Autodesk Inventor part; units mm, degrees
(part 2 of 2)
  spline S149 degree 2 poles (54.1022, 10.347) (54.1022, 11.4938) (55.3529, 12.7939) (56.4799, 12.7939) knots 0 0 0 1 2 2 2
  spline S150 degree 2 poles (56.4799, 12.7939) (57.607, 12.7939) (58.8527, 11.4889) (58.8527, 10.347) knots 0 0 0 1 2 2 2
  spline S151 degree 2 poles (57.3845, 10.3371) (57.3845, 10.7474) (57.2511, 11.2961) (57.1324, 11.4592) knots 0 0 0 1 2 2 2
  spline S152 degree 2 poles (57.1324, 11.4592) (57.0039, 11.6322) (56.6826, 11.7657) (56.4799, 11.7657) knots 0 0 0 1 2 2 2
  spline S153 degree 2 poles (56.4799, 11.7657) (56.2822, 11.7657) (55.9708, 11.6471) (55.8422, 11.479) knots 0 0 0 1 2 2 2
  spline S154 degree 2 poles (55.8422, 11.479) (55.7187, 11.3208) (55.5704, 10.7622) (55.5704, 10.3371) knots 0 0 0 1 2 2 2
  spline S155 degree 2 poles (55.5704, 10.3371) (55.5704, 9.9169) (55.7088, 9.3979) (55.8225, 9.2397) knots 0 0 0 1 2 2 2
  spline S156 degree 2 poles (55.8225, 9.2397) (55.9362, 9.0815) (56.2822, 8.9332) (56.4898, 8.9332) knots 0 0 0 1 2 2 2
  spline S157 degree 2 poles (56.4898, 8.9332) (56.6628, 8.9332) (57.0187, 9.0815) (57.1275, 9.2298) knots 0 0 0 1 2 2 2
  spline S158 degree 2 poles (57.1275, 9.2298) (57.2511, 9.4028) (57.3845, 9.9021) (57.3845, 10.3371) knots 0 0 0 1 2 2 2
  line L157 (63.9195, 8.0483) -> (62.4761, 8.0483)
  line L158 (62.4761, 8.0483) -> (62.4761, 10.3272)
  spline S159 degree 2 poles (62.4761, 10.3272) (62.4761, 10.609) (62.4316, 11.1626) (62.3723, 11.2911) knots 0 0 0 1 2 2 2
  spline S160 degree 2 poles (62.3723, 11.2911) (62.2982, 11.4493) (62.0213, 11.5828) (61.7841, 11.5828) knots 0 0 0 1 2 2 2
  spline S161 degree 2 poles (61.7841, 11.5828) (61.611, 11.5828) (61.2502, 11.4493) (61.0475, 11.306) knots 0 0 0 1 2 2 2
  line L159 (61.0475, 11.306) -> (61.0475, 8.0483)
  line L160 (61.0475, 8.0483) -> (59.614, 8.0483)
  line L161 (59.614, 8.0483) -> (59.614, 12.6505)
  line L162 (59.614, 12.6505) -> (61.0475, 12.6505)
  line L163 (61.0475, 12.6505) -> (61.0475, 12.1414)
  spline S162 degree 2 poles (61.0475, 12.1414) (61.3985, 12.438) (62.0658, 12.7741) (62.4712, 12.7741) knots 0 0 0 1 2 2 2
  spline S163 degree 2 poles (62.4712, 12.7741) (63.1731, 12.7741) (63.9195, 11.8843) (63.9195, 11.044) knots 0 0 0 1 2 2 2
  line L164 (63.9195, 11.044) -> (63.9195, 8.0483)
  spline S164 degree 2 poles (67.3403, 7.9248) (66.0353, 7.9248) (64.6462, 9.1705) (64.6462, 10.3223) knots 0 0 0 1 2 2 2
  spline S165 degree 2 poles (64.6462, 10.3223) (64.6462, 11.4493) (65.9413, 12.7939) (67.108, 12.7939) knots 0 0 0 1 2 2 2
  spline S166 degree 2 poles (67.108, 12.7939) (68.1609, 12.7939) (69.2286, 11.652) (69.2286, 10.5941) knots 0 0 0 1 2 2 2
  line L165 (69.2286, 10.5941) -> (69.2286, 10.0751)
  line L166 (69.2286, 10.0751) -> (66.0798, 10.0751)
  spline S167 degree 2 poles (66.0798, 10.0751) (66.0995, 9.7538) (66.3319, 9.3287) (66.5197, 9.2001) knots 0 0 0 1 2 2 2
  spline S168 degree 2 poles (66.5197, 9.2001) (66.7026, 9.0716) (67.1969, 8.9629) (67.4886, 8.9629) knots 0 0 0 1 2 2 2
  spline S169 degree 2 poles (67.4886, 8.9629) (67.7358, 8.9629) (68.2202, 9.0716) (68.4229, 9.1655) knots 0 0 0 1 2 2 2
  spline S170 degree 2 poles (68.4229, 9.1655) (68.6008, 9.2397) (68.8974, 9.4226) (68.9913, 9.4918) knots 0 0 0 1 2 2 2
  line L167 (68.9913, 9.4918) -> (69.1446, 9.4918)
  line L168 (69.1446, 9.4918) -> (69.1446, 8.3054)
  spline S171 degree 2 poles (69.1446, 8.3054) (68.9666, 8.2362) (68.6799, 8.1176) (68.4229, 8.0582) knots 0 0 0 1 2 2 2
  spline S172 degree 2 poles (68.4229, 8.0582) (68.1905, 7.994) (67.6962, 7.9248) (67.3403, 7.9248) knots 0 0 0 1 2 2 2
  spline S173 degree 2 poles (67.8148, 10.9402) (67.805, 11.3949) (67.4046, 11.8744) (66.9943, 11.8744) knots 0 0 0 1 2 2 2
  spline S174 degree 2 poles (66.9943, 11.8744) (66.5741, 11.8744) (66.0995, 11.3702) (66.0748, 10.9402) knots 0 0 0 1 2 2 2
  line L169 (66.0748, 10.9402) -> (67.8148, 10.9402)
  spline S175 degree 2 poles (71.3641, 7.9248) (70.8599, 7.9248) (69.9553, 8.1472) (69.6587, 8.2955) knots 0 0 0 1 2 2 2
  line L170 (69.6587, 8.2955) -> (69.6587, 9.5066)
  line L171 (69.6587, 9.5066) -> (69.7773, 9.5066)
  spline S176 degree 2 poles (69.7773, 9.5066) (69.8811, 9.4275) (70.1431, 9.2397) (70.3755, 9.1359) knots 0 0 0 1 2 2 2
  spline S177 degree 2 poles (70.3755, 9.1359) (70.5781, 9.0419) (71.0774, 8.9085) (71.374, 8.9085) knots 0 0 0 1 2 2 2
  spline S178 degree 2 poles (71.374, 8.9085) (71.6755, 8.9085) (72.1402, 9.0963) (72.1402, 9.299) knots 0 0 0 1 2 2 2
  spline S179 degree 2 poles (72.1402, 9.299) (72.1402, 9.4572) (71.9277, 9.6253) (71.6212, 9.6945) knots 0 0 0 1 2 2 2
  spline S180 degree 2 poles (71.6212, 9.6945) (71.458, 9.7389) (70.9588, 9.8329) (70.766, 9.8922) knots 0 0 0 1 2 2 2
  spline S181 degree 2 poles (70.766, 9.8922) (70.2222, 10.0603) (69.6785, 10.7177) (69.6785, 11.2565) knots 0 0 0 1 2 2 2
  spline S182 degree 2 poles (69.6785, 11.2565) (69.6785, 11.563) (69.9602, 12.1068) (70.2371, 12.3193) knots 0 0 0 1 2 2 2
  spline S183 degree 2 poles (70.2371, 12.3193) (70.5089, 12.527) (71.3147, 12.7741) (71.8238, 12.7741) knots 0 0 0 1 2 2 2
  spline S184 degree 2 poles (71.8238, 12.7741) (72.3083, 12.7741) (73.119, 12.5813) (73.3958, 12.4479) knots 0 0 0 1 2 2 2
  line L172 (73.3958, 12.4479) -> (73.3958, 11.2812)
  line L173 (73.3958, 11.2812) -> (73.2821, 11.2812)
  spline S185 degree 2 poles (73.2821, 11.2812) (73.208, 11.3406) (72.8866, 11.5334) (72.7384, 11.6026) knots 0 0 0 1 2 2 2
  spline S186 degree 2 poles (72.7384, 11.6026) (72.5554, 11.6817) (72.1106, 11.7904) (71.8782, 11.7904) knots 0 0 0 1 2 2 2
  spline S187 degree 2 poles (71.8782, 11.7904) (71.5668, 11.7904) (71.1367, 11.5778) (71.1367, 11.4048) knots 0 0 0 1 2 2 2
  spline S188 degree 2 poles (71.1367, 11.4048) (71.1367, 11.2466) (71.3493, 11.0687) (71.7052, 10.9797) knots 0 0 0 1 2 2 2
  spline S189 degree 2 poles (71.7052, 10.9797) (71.8881, 10.9352) (72.3676, 10.8512) (72.5901, 10.777) knots 0 0 0 1 2 2 2
  spline S190 degree 2 poles (72.5901, 10.777) (73.0844, 10.6189) (73.5985, 10.0009) (73.5985, 9.4868) knots 0 0 0 1 2 2 2
  spline S191 degree 2 poles (73.5985, 9.4868) (73.5985, 9.1655) (73.2969, 8.5773) (73.0152, 8.3795) knots 0 0 0 1 2 2 2
  spline S192 degree 2 poles (73.0152, 8.3795) (72.7235, 8.162) (71.9227, 7.9248) (71.3641, 7.9248) knots 0 0 0 1 2 2 2
  line L174 (75.7142, 8.0483) -> (74.2807, 8.0483)
  line L175 (74.2807, 8.0483) -> (74.2807, 12.6505)
  line L176 (74.2807, 12.6505) -> (75.7142, 12.6505)
  line L177 (75.7142, 12.6505) -> (75.7142, 8.0483)
  line L178 (75.7587, 13.308) -> (74.2411, 13.308)
  line L179 (74.2411, 13.308) -> (74.2411, 14.4252)
  line L180 (74.2411, 14.4252) -> (75.7587, 14.4252)
  line L181 (75.7587, 14.4252) -> (75.7587, 13.308)
  spline S193 degree 2 poles (79.3475, 8.5377) (79.1992, 8.4142) (78.9669, 8.2164) (78.7691, 8.1176) knots 0 0 0 1 2 2 2
  spline S194 degree 2 poles (78.7691, 8.1176) (78.5764, 8.0236) (78.2106, 7.9248) (77.8843, 7.9248) knots 0 0 0 1 2 2 2
  spline S195 degree 2 poles (77.8843, 7.9248) (77.2713, 7.9248) (76.4656, 8.7453) (76.4656, 9.3682) knots 0 0 0 1 2 2 2
  spline S196 degree 2 poles (76.4656, 9.3682) (76.4656, 9.8774) (76.8759, 10.5101) (77.2614, 10.693) knots 0 0 0 1 2 2 2
  spline S197 degree 2 poles (77.2614, 10.693) (77.652, 10.8808) (78.7345, 11.0291) (79.3574, 11.0687) knots 0 0 0 1 2 2 2
  line L182 (79.3574, 11.0687) -> (79.3574, 11.0934)
  spline S198 degree 2 poles (79.3574, 11.0934) (79.3574, 11.474) (78.7939, 11.7657) (78.2303, 11.7657) knots 0 0 0 1 2 2 2
  spline S199 degree 2 poles (78.2303, 11.7657) (77.9782, 11.7657) (77.296, 11.5828) (76.9747, 11.4394) knots 0 0 0 1 2 2 2
  line L183 (76.9747, 11.4394) -> (76.8512, 11.4394)
  line L184 (76.8512, 11.4394) -> (76.8512, 12.5517)
  spline S200 degree 2 poles (76.8512, 12.5517) (77.0637, 12.611) (78.0128, 12.7791) (78.4973, 12.7791) knots 0 0 0 1 2 2 2
  spline S201 degree 2 poles (78.4973, 12.7791) (79.6837, 12.7791) (80.7712, 11.9881) (80.7712, 11.1774) knots 0 0 0 1 2 2 2
  line L185 (80.7712, 11.1774) -> (80.7712, 8.0483)
  line L186 (80.7712, 8.0483) -> (79.3475, 8.0483)
  line L187 (79.3475, 8.0483) -> (79.3475, 8.5377)
  line L188 (79.3475, 9.2496) -> (79.3475, 10.2036)
  spline S202 degree 2 poles (79.3475, 10.2036) (78.9817, 10.169) (78.5319, 10.1146) (78.3144, 10.0355) knots 0 0 0 1 2 2 2
  spline S203 degree 2 poles (78.3144, 10.0355) (78.1216, 9.9713) (77.914, 9.7043) (77.914, 9.4868) knots 0 0 0 1 2 2 2
  spline S204 degree 2 poles (77.914, 9.4868) (77.914, 9.1655) (78.2649, 8.9233) (78.606, 8.9233) knots 0 0 0 1 2 2 2
  spline S205 degree 2 poles (78.606, 8.9233) (78.7939, 8.9233) (79.1893, 9.0963) (79.3475, 9.2496) knots 0 0 0 1 2 2 2
  point P0 (60.406, 3)
  constraints: 2 other
extrude "Extrusion36" cut sketch "Sketch38" against normal blind 2
equation "\"d249\" = 0.5 * d248"
equation "\"d243\" = 0.5 * d242"
equation "\"d255\" = d254"
body "Solid2"
